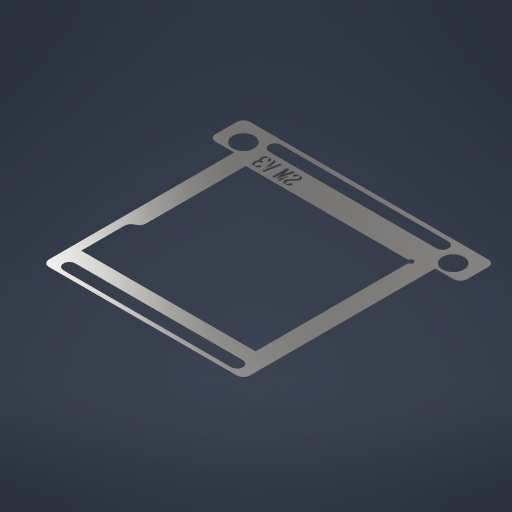
# Autodesk Inventor part: Sensor Mount Film Stencil - V1
Saved by Autodesk Inventor 2024 (Build 280153000, 153)
## iProperties
Created: 2022-06-23
Part Number: Sensor Mount Film Stencil - V1
Material: Stainless Steel
Document SubType Name: Modeling
Designer: Caleb
Density: 8 g/cm^3
Appearance: Semi-Polished
Author: Caleb
Autodesk Inventor part; units mm, degrees
ref_plane "YZ Plane" through (0, 0, 0) normal (1, 0, 0) x (0, 1, 0)
ref_plane "XZ Plane" through (0, 0, 0) normal (0, 1, 0) x (-1, 0, 0)
ref_plane "XY Plane" through (0, 0, 0) normal (0, 0, 1) x (1, 0, 0)
sketch "Sketch1" plane through (0, 0, 0) normal (0, 1, 0) x (-1, 0, 0)
  line L0 (-38.1, -34.29) -> (38.1, -34.29)
  line L1 (38.1, -34.29) -> (38.1, 34.29)
  line L2 (38.1, 34.29) -> (-38.1, 34.29)
  line L3 (-38.1, 34.29) -> (-38.1, -34.29)
  line L4 (-38.1, -34.29) -> (38.1, 34.29) construction
  line L5 (38.1, -34.29) -> (-38.1, 34.29) construction
  point P0 (0, 0)
  dimension "d0" = 76.2
  dimension "d1" = 68.58
  constraints: 12 end point, 2 midpoint, 2 parallel, 1 horizontal, 1 perpendicular
  measures "d0" distance of L2.end L1.end
  measures "d1" distance of L1.end L0.end
extrude "Extrusion1" add sketch "Sketch1" along normal blind 0.0508
sketch "Sketch2" plane through (0, 0.0508, 0) normal (0, 1, 0) x (1, 0, 0)
  line L0 (-38.1, -34.29) -> (38.1, -34.29) projected
  line L1 (-46.3971, 0) -> (43.7494, 0)
  line L2 (-38.1, 34.29) -> (-38.1, -34.29) projected
  line L3 (38.1, -34.29) -> (38.1, 34.29) projected
  line L4 (38.1, 23.79) -> (30.48, 23.79)
  line L5 (30.48, 23.79) -> (30.48, -34.29)
  line L6 (30.48, -34.29) -> (38.1, -34.29)
  line L7 (38.1, -34.29) -> (38.1, 23.79)
  line L8 (0, -45.6355) -> (0, 71.8702)
  line L9 (46.3971, 0) -> (-43.7494, 0)
  line L10 (-38.1, -34.29) -> (-38.1, 34.29)
  line L11 (-38.1, 23.79) -> (-30.48, 23.79)
  line L12 (-30.48, 23.79) -> (-30.48, -34.29)
  line L13 (-30.48, -34.29) -> (-38.1, -34.29)
  line L14 (-38.1, -34.29) -> (-38.1, 23.79)
  line L15 (38.1, 34.29) -> (-38.1, 34.29) projected
  point P0 (0, 0)
  point P1 (38.1, -31.05)
  dimension "d14" = 7.62
  dimension "d16" = 10.5
  constraints: 24 end point, 6 symmetric about line, 3 point on line, 2 horizontal, 2 parallel, 1 perpendicular, 1 vertical
  measures "d14" distance of L5.end L6.end
  measures "d16" distance between parallel lines of L15 L4
extrude "Extrusion2" cut sketch "Sketch2" against normal through all contours L2 L1 L12 L0 | L2 L11 L12 L1 | L5 L1 L3 L0 | L5 L4 L3 L1
sketch "Sketch3" plane through (0, 0.0508, 0) normal (0, 1, 0) x (1, 0, 0)
  line L0 (25.4, -31.115) -> (-25.4, -31.115) construction
  line L1 (25.4, -29.365) -> (-25.4, -29.365)
  line L2 (-25.4, -32.865) -> (25.4, -32.865)
  arc A0 (25.4, -32.865) -> (25.4, -29.365) centre (25.4, -31.115) ccw
  arc A1 (-25.4, -29.365) -> (-25.4, -32.865) centre (-25.4, -31.115) ccw
  line L3 (25.4, 31.115) -> (-25.4, 31.115) construction
  line L4 (25.4, 32.865) -> (-25.4, 32.865)
  line L5 (-25.4, 29.365) -> (25.4, 29.365)
  arc A2 (25.4, 29.365) -> (25.4, 32.865) centre (25.4, 31.115) ccw
  arc A3 (-25.4, 32.865) -> (-25.4, 29.365) centre (-25.4, 31.115) ccw
  line L6 (38.1, 34.29) -> (-38.1, 34.29) projected
  line L7 (-38.1, -34.29) -> (38.1, -34.29) projected
  point P0 (0, 0)
  point P1 (0, -31.115)
  point P2 (0, 31.115)
  dimension "d17" = 3.5
  dimension "d18" = 3.5
  dimension "d19" = 50.8
  dimension "d20" = 50.8
  dimension "d21" = 3.175
  dimension "d22" = 3.175
  constraints: 16 end point, 8 point on circle, 8 tangent, 4 centre point, 3 parallel, 2 midpoint, 2 vertical alignment, 1 horizontal
  measures "d17" distance between parallel lines of L2 L1
  measures "d18" distance between parallel lines of L4 L5
  measures "d19" distance of L0.end L0.start
  measures "d20" distance of L3.end L3.start
  measures "d21" distance from line of L6 point (0, 31.115)
  measures "d22" distance from line of L7 point (0, -31.115)
extrude "Extrusion3" cut sketch "Sketch3" against normal through all
sketch "Sketch6" plane through (0, 0.0508, 0) normal (0, 1, 0) x (1, 0, 0)
  line L0 (38.1, 34.29) -> (-38.1, 34.29) projected
  line L1 (-38.1, 34.29) -> (-38.1, 23.79) projected
  line L2 (38.1, 23.79) -> (38.1, 34.29) projected
  point P0 (0, 0)
  point P1 (-31.75, 27.94)
  point P2 (31.75, 27.94)
  dimension "d41" = 6.35
  dimension "d42" = 6.35
  dimension "d43" = 6.35
  constraints: 1 horizontal alignment
  measures "d41" distance from line of L0 point (-31.75, 27.94)
  measures "d42" distance from line of L1 point (-31.75, 27.94)
  measures "d43" distance from line of point (31.75, 27.94) L2
hole "Hole1" at (-31.75, 0.0508, -27.94) at (31.75, 0.0508, -27.94) direction (0, -1, 0) diameter 6.477 end through all
sketch "Sketch4" plane through (0, 0.0508, 0) normal (0, 1, 0) x (1, 0, 0)
  line L0 (-25.105, -25.025) -> (24.895, -25.025)
  line L1 (24.895, -25.025) -> (24.895, 21.975)
  line L2 (24.895, 21.975) -> (-25.105, 21.975)
  line L3 (-25.105, 21.975) -> (-25.105, -25.025)
  line L4 (38.1, 34.29) -> (-38.1, 34.29) projected
  line L5 (38.1, 23.79) -> (38.1, 34.29) projected
  circle A0 centre (24.895, 21.975) radius 0.7938
  circle A1 centre (31.75, 27.94) radius 3.2385 projected
  point P0 (0, 0)
  point P1 (24.895, 21.1813)
  point P2 (24.1012, 21.975)
  point P3 (29.845, 22.225)
  dimension "d29" = 1.5875
  dimension "d39" = 47
  dimension "d40" = 50
  dimension "d52" = 1.905
  dimension "d53" = 5.715
  dimension "d54" = 0.25
  dimension "d55" = 4.95
  constraints: 8 end point, 2 parallel, 1 centre point, 1 coincident, 1 horizontal, 1 perpendicular
  measures "d29" diameter of A0
  measures "d39" distance of L2.end L0.start
  measures "d40" distance of L1.end L2.end
  measures "d52" horizontal distance of point (29.845, 22.225) A1.centre
  measures "d53" vertical distance of point (29.845, 22.225) A1.centre
  measures "d54" distance from line of L2 point (29.845, 22.225)
  measures "d55" distance from line of L1 point (29.845, 22.225)
extrude "Extrusion4" cut sketch "Sketch4" against normal through all contours L3 L2 A0 L1 L0 | A0 L2 L1 | L1 L2 A0
sketch "Sketch5" plane through (0, 0.0508, 0) normal (0, 1, 0) x (1, 0, 0)
  line L0 (-25.105, 21.975) -> (-25.105, -25.025) projected
  line L1 (-25.105, -25.025) -> (-27.7925, -25.025)
  line L2 (-27.7925, -25.025) -> (-27.7925, -10.025)
  line L3 (-27.7925, -10.025) -> (-25.105, -10.025)
  line L4 (-25.105, -10.025) -> (-25.105, -25.025)
  line L5 (-30.48, 23.79) -> (-30.48, -34.29) projected
  point P0 (0, 0)
  point P1 (-30.48, -31.05)
  point P2 (-25.105, -10.025)
  dimension "d30" = 15
  dimension "d31" = 5.375
  dimension "d32" = 2.6875
  constraints: 8 end point, 2 parallel, 1 horizontal, 1 perpendicular
  measures "d30" distance of L1.end L2.end
  measures "d31" distance between parallel lines of L5 L0
  measures "d32" distance of L2.end L3.end
extrude "Extrusion5" cut sketch "Sketch5" against normal through all
fillet "Fillet1" radius 2 8 edges at (-38.1, 0.0254, -34.29) (38.1, 0.0254, -34.29) (38.1, 0.0254, -23.79) (-38.1, 0.0254, -23.79) (30.48, 0.0254, 34.29) (-30.48, 0.0254, 34.29) (-25.105, 0.0254, 10.025) (-27.7925, 0.0254, 10.025)
sketch "Sketch8" plane through (0, 0, 0) normal (0, -1, 0) x (1, 0, 0)
  line L0 (-12.9863, -27.7999) -> (-28.0129, -27.7999) construction
  line L1 (-28.0129, -27.7999) -> (-28.0129, -23.9751) construction
  line L2 (-28.0129, -23.9751) -> (-12.9863, -23.9751) construction
  line L3 (-12.9863, -23.9751) -> (-12.9863, -27.7999) construction
  spline S0 degree 2 poles (-14.105, -25.4183) (-14.2429, -25.2773) (-14.5061, -25.0047) (-14.622, -24.8793) knots 0 0 0 1 2 2 2
  spline S1 degree 2 poles (-14.622, -24.8793) (-14.7881, -24.7038) (-14.9762, -24.3967) (-14.9762, -24.2777) knots 0 0 0 1 2 2 2
  spline S2 degree 2 poles (-14.9762, -24.2777) (-14.973, -24.1116) (-14.7787, -23.8546) (-14.622, -23.7888) knots 0 0 0 1 2 2 2
  line L4 (-14.622, -23.7888) -> (-14.622, -23.2749)
  spline S3 degree 2 poles (-14.622, -23.2749) (-15.0012, -23.3532) (-15.4838, -23.8734) (-15.4963, -24.2432) knots 0 0 0 1 2 2 2
  spline S4 degree 2 poles (-15.4963, -24.2432) (-15.4963, -24.4312) (-15.2457, -24.8668) (-14.8477, -25.3368) (-14.622, -25.5719) knots 0 0 0 1 2 3 3 3
  spline S5 degree 2 poles (-14.622, -25.5719) (-14.4842, -25.7223) (-14.2209, -26.0075) (-14.105, -26.1453) knots 0 0 0 1 2 2 2
  spline S6 degree 2 poles (-14.105, -26.1453) (-13.9483, -26.3271) (-13.7571, -26.6499) (-13.7509, -26.7783) knots 0 0 0 1 2 2 2
  spline S7 degree 2 poles (-13.7509, -26.7783) (-13.7477, -26.935) (-13.9452, -27.1983) (-14.105, -27.2672) knots 0 0 0 1 2 2 2
  line L5 (-14.105, -27.2672) -> (-14.105, -27.7341)
  spline S8 degree 2 poles (-14.105, -27.7341) (-13.8543, -27.6809) (-13.4626, -27.4051) (-13.2338, -27.0071) (-13.2307, -26.7658) knots 0 0 0 1 2 3 3 3
  spline S9 degree 2 poles (-13.2307, -26.7658) (-13.2369, -26.559) (-13.4876, -26.1077) (-13.8825, -25.6439) (-14.105, -25.4183) knots 0 0 0 1 2 3 3 3
  spline S10 degree 2 poles (-13.2307, -24.2432) (-13.2432, -23.8859) (-13.7258, -23.3595) (-14.105, -23.2749) knots 0 0 0 1 2 2 2
  line L6 (-14.105, -23.2749) -> (-14.105, -23.7888)
  spline S11 degree 2 poles (-14.105, -23.7888) (-13.9483, -23.8546) (-13.754, -24.1147) (-13.7509, -24.2777) knots 0 0 0 1 2 2 2
  spline S12 degree 2 poles (-13.7509, -24.2777) (-13.7477, -24.3717) (-13.6161, -24.4155) (-13.5378, -24.4124) knots 0 0 0 1 2 2 2
  line L7 (-13.5378, -24.4124) -> (-13.4563, -24.4124)
  spline S13 degree 2 poles (-13.4563, -24.4124) (-13.3529, -24.4155) (-13.2338, -24.3529) (-13.2307, -24.2432) knots 0 0 0 1 2 2 2
  spline S14 degree 2 poles (-14.622, -27.2672) (-14.7787, -27.2014) (-14.973, -26.9413) (-14.9762, -26.7783) knots 0 0 0 1 2 2 2
  spline S15 degree 2 poles (-14.9762, -26.7783) (-14.9793, -26.6467) (-15.1203, -26.5872) (-15.208, -26.5935) knots 0 0 0 1 2 2 2
  line L8 (-15.208, -26.5935) -> (-15.2895, -26.5935)
  spline S16 degree 2 poles (-15.2895, -26.5935) (-15.3428, -26.5872) (-15.4901, -26.6467) (-15.4963, -26.7658) knots 0 0 0 1 2 2 2
  spline S17 degree 2 poles (-15.4963, -26.7658) (-15.4932, -27.004) (-15.2645, -27.402) (-14.8727, -27.6809) (-14.622, -27.7341) knots 0 0 0 1 2 3 3 3
  line L9 (-14.622, -27.7341) -> (-14.622, -27.2672)
  line L10 (-16.5743, -25.6753) -> (-16.5743, -25.6941)
  line L11 (-16.5743, -25.6941) -> (-17.1729, -23.4817)
  line L12 (-17.1729, -23.4817) -> (-17.762, -25.7129)
  line L13 (-17.762, -25.7129) -> (-17.7683, -23.488)
  spline S18 degree 2 poles (-17.7683, -23.488) (-17.7683, -23.3939) (-17.8874, -23.2811) (-17.9939, -23.2749) knots 0 0 0 1 2 2 2
  line L14 (-17.9939, -23.2749) -> (-18.0503, -23.2749)
  spline S19 degree 2 poles (-18.0503, -23.2749) (-18.1631, -23.278) (-18.2885, -23.4002) (-18.2885, -23.4942) knots 0 0 0 1 2 2 2
  line L15 (-18.2885, -23.4942) -> (-18.2885, -27.5555)
  spline S20 degree 2 poles (-18.2885, -27.5555) (-18.2822, -27.6621) (-18.1349, -27.7749) (-18.019, -27.7749) knots 0 0 0 1 2 2 2
  line L16 (-18.019, -27.7749) -> (-17.9688, -27.7749)
  spline S21 degree 2 poles (-17.9688, -27.7749) (-17.8686, -27.7686) (-17.7307, -27.6746) (-17.7056, -27.5868) knots 0 0 0 1 2 2 2
  line L17 (-17.7056, -27.5868) -> (-17.1635, -25.4246)
  line L18 (-17.1635, -25.4246) -> (-16.6245, -27.5931)
  spline S22 degree 2 poles (-16.6245, -27.5931) (-16.5963, -27.6715) (-16.4741, -27.7592) (-16.3832, -27.7749) knots 0 0 0 1 2 2 2
  line L19 (-16.3832, -27.7749) -> (-16.239, -27.7749)
  spline S23 degree 2 poles (-16.239, -27.7749) (-16.1576, -27.7561) (-16.0635, -27.6683) (-16.0541, -27.5994) knots 0 0 0 1 2 2 2
  line L20 (-16.0541, -27.5994) -> (-16.5743, -25.6753)
  spline S24 degree 2 poles (-16.0479, -23.5193) (-16.0479, -23.419) (-16.1638, -23.278) (-16.2798, -23.2749) knots 0 0 0 1 2 2 2
  line L21 (-16.2798, -23.2749) -> (-16.3174, -23.2749)
  spline S25 degree 2 poles (-16.3174, -23.2749) (-16.3268, -23.2749) (-16.3362, -23.2749) knots 0 0 0 1 1 1
  spline S26 degree 2 poles (-16.3362, -23.2749) (-16.4427, -23.278) (-16.5681, -23.4159) (-16.5681, -23.5193) knots 0 0 0 1 2 2 2
  line L22 (-16.5681, -23.5193) -> (-16.5681, -23.7763)
  line L23 (-16.5681, -23.7763) -> (-16.0479, -25.7004)
  line L24 (-16.0479, -25.7004) -> (-16.0479, -23.5193)
  line L25 (-20.0214, -27.6965) -> (-20.855, -23.3783)
  spline S27 degree 2 poles (-20.855, -23.3783) (-20.8769, -23.3031) (-20.9459, -23.2717) (-20.996, -23.2749) knots 0 0 0 1 2 2 2
  line L26 (-20.996, -23.2749) -> (-21.2812, -23.2749)
  spline S28 degree 2 poles (-21.2812, -23.2749) (-21.3125, -23.2749) (-21.3564, -23.2811) (-21.3752, -23.2937) knots 0 0 0 1 2 2 2
  line L27 (-21.3752, -23.2937) -> (-20.8613, -26.0169)
  line L28 (-20.8613, -26.0169) -> (-20.5353, -27.7091)
  spline S29 degree 2 poles (-20.5353, -27.7091) (-20.5259, -27.7592) (-20.4852, -27.7905) (-20.4382, -27.7937) knots 0 0 0 1 2 2 2
  line L29 (-20.4382, -27.7937) -> (-20.1186, -27.7937)
  spline S30 degree 2 poles (-20.1186, -27.7937) (-20.0653, -27.7937) (-20.012, -27.7529) (-20.0214, -27.6965) knots 0 0 0 1 2 2 2
  line L30 (-21.6447, -24.5973) -> (-22.2432, -27.684)
  spline S31 degree 2 poles (-22.2432, -27.684) (-22.2526, -27.7467) (-22.215, -27.7937) (-22.1711, -27.7937) knots 0 0 0 1 2 2 2
  line L31 (-22.1711, -27.7937) -> (-21.8515, -27.7937)
  spline S32 degree 2 poles (-21.8515, -27.7937) (-21.8076, -27.7937) (-21.745, -27.7529) (-21.7293, -27.6903) knots 0 0 0 1 2 2 2
  line L32 (-21.7293, -27.6903) -> (-21.394, -25.9511)
  line L33 (-21.394, -25.9511) -> (-21.6447, -24.5973)
  spline S33 degree 2 poles (-23.8257, -25.3024) (-23.9824, -25.3024) (-24.2613, -25.1676) (-24.4399, -24.9232) (-24.4431, -24.7634) knots 0 0 0 1 2 3 3 3
  line L34 (-24.4431, -24.7634) -> (-24.4431, -24.2338)
  spline S34 degree 2 poles (-24.4431, -24.2338) (-24.4399, -24.0708) (-24.2457, -23.8107) (-24.0827, -23.7449) knots 0 0 0 1 2 2 2
  line L35 (-24.0827, -23.7449) -> (-24.0827, -23.2749)
  spline S35 degree 2 poles (-24.0827, -23.2749) (-24.3397, -23.3281) (-24.7314, -23.6133) (-24.9539, -24.0176) (-24.957, -24.2463) knots 0 0 0 1 2 3 3 3
  line L36 (-24.957, -24.2463) -> (-24.957, -24.7477)
  spline S36 degree 2 poles (-24.957, -24.7477) (-24.9539, -24.9827) (-24.7251, -25.3933) (-24.5214, -25.5405) knots 0 0 0 1 2 2 2
  spline S37 degree 2 poles (-24.5214, -25.5405) (-24.7251, -25.6847) (-24.9539, -26.0952) (-24.957, -26.324) knots 0 0 0 1 2 2 2
  line L37 (-24.957, -26.324) -> (-24.957, -26.8316)
  spline S38 degree 2 poles (-24.957, -26.8316) (-24.9539, -27.0604) (-24.7251, -27.4584) (-24.3334, -27.7435) (-24.0827, -27.7999) knots 0 0 0 1 2 3 3 3
  line L38 (-24.0827, -27.7999) -> (-24.0827, -27.333)
  spline S39 degree 2 poles (-24.0827, -27.333) (-24.2457, -27.2609) (-24.4399, -27.004) (-24.4431, -26.8379) knots 0 0 0 1 2 2 2
  line L39 (-24.4431, -26.8379) -> (-24.4431, -26.3114)
  spline S40 degree 2 poles (-24.4431, -26.3114) (-24.4399, -26.1485) (-24.2582, -25.9072) (-23.9793, -25.7724) (-23.8257, -25.7724) knots 0 0 0 1 2 3 3 3
  spline S41 degree 2 poles (-23.8257, -25.7724) (-23.669, -25.7724) (-23.5656, -25.7192) (-23.5719, -25.6565) knots 0 0 0 1 2 2 2
  line L40 (-23.5719, -25.6565) -> (-23.5719, -25.5405)
  spline S42 degree 2 poles (-23.5719, -25.5405) (-23.5688, -25.4653) (-23.5719, -25.3588) (-23.6785, -25.3024) (-23.8257, -25.3024) knots 0 0 0 1 2 3 3 3
  line L41 (-22.6976, -26.9068) -> (-22.6976, -26.8316)
  spline S43 degree 2 poles (-22.6976, -26.8316) (-22.6945, -26.7251) (-22.754, -26.6655) (-22.8512, -26.6718) knots 0 0 0 1 2 2 2
  spline S44 degree 2 poles (-22.8512, -26.6718) (-22.8762, -26.6718) (-22.9264, -26.6718) (-22.9546, -26.6718) knots 0 0 0 1 2 2 2
  spline S45 degree 2 poles (-22.9546, -26.6718) (-23.0016, -26.6718) (-23.0329, -26.6718) knots 0 0 0 1 1 1
  spline S46 degree 2 poles (-23.0329, -26.6718) (-23.152, -26.6655) (-23.2178, -26.7251) (-23.2178, -26.8379) knots 0 0 0 1 2 2 2
  spline S47 degree 2 poles (-23.2178, -26.8379) (-23.2209, -27.004) (-23.409, -27.2609) (-23.5719, -27.333) knots 0 0 0 1 2 2 2
  line L42 (-23.5719, -27.333) -> (-23.5719, -27.7999)
  spline S48 degree 2 poles (-23.5719, -27.7999) (-23.2084, -27.7153) (-22.7321, -27.2327) (-22.6976, -26.9068) knots 0 0 0 1 2 2 2
  spline S49 degree 2 poles (-23.5782, -23.2749) (-23.5719, -23.2843) (-23.5719, -23.3031) (-23.5719, -23.3125) knots 0 0 0 1 2 2 2
  line L43 (-23.5719, -23.3125) -> (-23.5719, -23.7512)
  spline S50 degree 2 poles (-23.5719, -23.7512) (-23.409, -23.8139) (-23.2209, -24.0708) (-23.2178, -24.2369) knots 0 0 0 1 2 2 2
  spline S51 degree 2 poles (-23.2178, -24.2369) (-23.2209, -24.3435) (-23.1739, -24.4093) (-23.0956, -24.403) knots 0 0 0 1 2 2 2
  spline S52 degree 2 poles (-23.0956, -24.403) (-23.0486, -24.403) (-22.9608, -24.403) knots 0 0 0 1 1 1
  spline S53 degree 2 poles (-22.9608, -24.403) (-22.9232, -24.403) (-22.8606, -24.403) (-22.8324, -24.403) knots 0 0 0 1 2 2 2
  spline S54 degree 2 poles (-22.8324, -24.403) (-22.7477, -24.4093) (-22.6945, -24.3529) (-22.6976, -24.2494) knots 0 0 0 1 2 2 2
  spline S55 degree 2 poles (-22.6976, -24.2494) (-22.7007, -24.0207) (-22.9232, -23.6196) (-23.3181, -23.3313) (-23.5782, -23.2749) knots 0 0 0 1 2 3 3 3
  point P0 (0, 0)
  dimension "d0" = 76.2
  dimension "d1" = 68.58
  constraints: 2 other
emboss "Emboss2" sketch "Sketch8" operation cut depth 1 direction (0, 1, 0)
equation "\"d18\" = d17"
equation "\"d20\" = d19"
equation "\"d43\" = d42"
equation "\"d32\" = 0.5 * d31"
body "Solid1"
